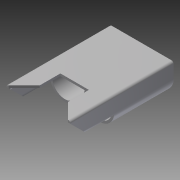
# Autodesk Inventor part: FuseHolder
Saved by Autodesk Inventor 2014 SP1 (Build 180222100, 222)
## iProperties
Created: 2016-03-18
Part Number: FuseHolder
Material: Steel
Document SubType Name: Modeling
Designer: Tyler
Density: 7.85 g/cm^3
Appearance: Steel
Author: Tyler
Autodesk Inventor part; units mm, degrees
ref_plane "YZ Plane" through (0, 0, 0) normal (1, 0, 0) x (0, 1, 0)
ref_plane "XZ Plane" through (0, 0, 0) normal (0, 1, 0) x (-1, 0, 0)
ref_plane "XY Plane" through (0, 0, 0) normal (0, 0, 1) x (1, 0, 0)
sketch "Sketch1" plane through (0, 0, 0) normal (0, 1, 0) x (-1, 0, 0)
  line L0 (0, 3.2) -> (-3.2, 3.2)
  line L1 (-3.45, 2.95) -> (-3.45, 1.6)
  arc A0 (-3.45, 1.6) -> (-0.3045, 2.0141) centre (-1.85, 1.6) ccw
  line L2 (0, 0) -> (-5.7029, 0) construction
  line L3 (-1.85, 1.6) -> (-0.3045, 2.0141) construction
  line L4 (0, 2.95) -> (-2.95, 2.95)
  line L5 (-3.2, 2.7) -> (-3.2, 1.6)
  arc A1 (-3.2, 1.6) -> (-0.5038, 1.7019) centre (-1.85, 1.6) ccw
  line L6 (-0.5038, 1.7019) -> (-1.7853, 1.3585) construction
  line L7 (-0.5038, 1.7019) -> (-0.3045, 2.0141)
  line L8 (0, 0) -> (0, 1.4199) construction
  line L9 (0, 3.2) -> (3.2, 3.2)
  line L10 (3.45, 2.95) -> (3.45, 1.6)
  arc A2 (0.3045, 2.0141) -> (3.45, 1.6) centre (1.85, 1.6) ccw
  line L11 (0, 0) -> (5.7029, 0) construction
  line L12 (1.85, 1.6) -> (0.3045, 2.0141) construction
  line L13 (0, 2.95) -> (2.95, 2.95)
  line L14 (3.2, 2.7) -> (3.2, 1.6)
  arc A3 (0.5038, 1.7019) -> (3.2, 1.6) centre (1.85, 1.6) ccw
  line L15 (0.5038, 1.7019) -> (1.7853, 1.3585) construction
  line L16 (0.5038, 1.7019) -> (0.3045, 2.0141)
  arc A4 (-3.2, 3.2) -> (-3.45, 2.95) centre (-3.2, 2.95) ccw
  arc A5 (-2.95, 2.95) -> (-3.2, 2.7) centre (-2.95, 2.7) ccw
  arc A6 (3.2, 2.7) -> (2.95, 2.95) centre (2.95, 2.7) ccw
  arc A7 (3.45, 2.95) -> (3.2, 3.2) centre (3.2, 2.95) ccw
  point P0 (-3.45, 3.2)
  point P1 (-3.2, 2.95)
  point P2 (3.45, 3.2)
  point P3 (3.2, 2.95)
  dimension "d0" = 3.45
  dimension "d1" = 0
  dimension "d2" = 3.2
  dimension "d3" = 15
  dimension "d4" = 1.6
  dimension "d5" = 1.6
  dimension "d6" = 0.25
  dimension "d9" = 0.25
  dimension "d10" = 0.25
  dimension "d11" = 0.25
  dimension "d12" = 0.25
  constraints: 34 end point, 16 point on circle, 10 tangent, 9 symmetric about line, 8 centre point, 8 point on line, 3 perpendicular, 1 horizontal, 1 parallel, 5 other
  measures "d0" distance from line of L2.start L1
  measures "d1" horizontal distance of L2.start L0.start
  measures "d2" distance from line of L2.start L0
  measures "d3" angle of L3 L2
  measures "d4" radius of A0
  measures "d5" distance of point (-3.45, 3.2) L1.end
  measures "d6" distance between parallel lines of L0 L4
  measures "d9" radius of A4
  measures "d10" radius of A5
  measures "d11" radius of A6
  measures "d12" radius of A7
extrude "Extrusion1" add sketch "Sketch1" along normal blind 11.1
sketch "Sketch2" plane through (-3.2, 0, 3.2) normal (0, 0, 1) x (1, 0, 0)
  line L0 (0, 0) -> (6.4, 0) projected
  line L1 (0, 11.1) -> (6.4, 11.1) projected
  line L2 (0, 0) -> (0, 11.1) projected
  line L3 (3.2, 0) -> (3.2, 8.5352) construction
  line L4 (3.2, 3.9) -> (1.67, 3.9)
  line L5 (1.67, 3.9) -> (1.67, 1.67)
  line L6 (1.67, 1.67) -> (0, 0)
  line L7 (-0.25, 0) -> (-0.25, 11.1) projected
  line L8 (3.2, 3.9) -> (4.73, 3.9)
  line L9 (4.73, 3.9) -> (4.73, 1.67)
  line L10 (4.73, 1.67) -> (6.4, 0)
  dimension "d27" = 7.2
  dimension "d28" = 45
  dimension "d29" = 1.92
  dimension "d30" = 1.53
  constraints: 14 end point, 2 perpendicular, 2 symmetric about line, 1 parallel, 1 point on line
  measures "d27" distance between parallel lines of L4 L1
  measures "d28" angle of L5 L6
  measures "d29" distance between parallel lines of L7 L5
  measures "d30" distance of L4.start L4.end
sketch "Sketch3" plane through (3.45, 0, 2.95) normal (1, 0, 0) x (0, 0, -1)
  line L0 (0, 0) -> (0, 11.1) projected
  line L1 (6.53, 4.7) -> (1.53, 4.7)
  line L2 (1.53, 4.7) -> (1.53, 1.53)
  line L3 (1.53, 1.53) -> (0, 0)
  line L4 (6.53, 4.7) -> (6.53, -3)
  line L5 (6.53, -3) -> (0, -3)
  line L6 (0, -3) -> (0, 0)
  line L7 (2.95, 11.1) -> (0.9359, 11.1) projected
  line L8 (-0.25, 0) -> (-0.25, 11.1) projected
  point P0 (2.95, 0)
  dimension "d13" = 6.4
  dimension "d14" = 1.78
  dimension "d15" = 45
  dimension "d16" = 3
  dimension "d17" = 5
  constraints: 12 end point, 3 perpendicular, 1 collinear, 1 parallel
  measures "d13" distance between parallel lines of L1 L7
  measures "d14" distance between parallel lines of L8 L2
  measures "d15" angle of L2 L3
  measures "d16" distance of L5.end L0.start
  measures "d17" distance of L1.start L1.end
extrude "Extrusion2" cut sketch "Sketch3" against normal through all
sketch "Sketch4" plane through (-0.2602, 4.7, 1.42) normal (0, 0, -1) x (-1, 0, 0)
  line L0 (-1.0096, -4.7) -> (0.4904, -4.7)
  line L1 (0.4904, -4.7) -> (0.4904, 0.8)
  line L2 (0.4904, 0.8) -> (-1.0096, 0.8)
  line L3 (-1.0096, 0.8) -> (-1.0096, -4.7)
  line L4 (-1.0096, -4.7) -> (0.4904, 0.8) construction
  line L5 (0.4904, -4.7) -> (-1.0096, 0.8) construction
  point P0 (-0.2602, -4.7)
  point P1 (-0.2596, -1.95)
  dimension "d20" = 1.5
  dimension "d21" = 0
  dimension "d22" = 5.5
  constraints: 12 end point, 2 midpoint, 2 parallel, 1 horizontal, 1 perpendicular
  measures "d20" distance of L0.start L0.end
  measures "d21" distance from line of point (-0.26, -4.7) L0
  measures "d22" distance of L0.end L1.end
extrude "Extrusion3" cut sketch "Sketch4" along normal blind 11.1 and the other way blind 1
extrude "Extrusion4" cut sketch "Sketch2" against normal through all
equation "\"d4\" = d5"
body "Solid1"
